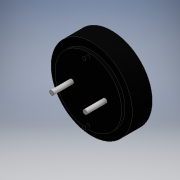
# Autodesk Inventor part: BUZZER_TDK_PS12
Saved by Autodesk Inventor 2016 (Build 200138000, 138)
## iProperties
Created: 2018-08-01
Part Number: BUZZER_TDK_PS12
Material: Generic
Document SubType Name: Modeling
Designer: Luke
Density: 1 g/cm^3
Appearance: Default
Author: Luke
Autodesk Inventor part; units mm, degrees
ref_plane "YZ Plane" through (0, 0, 0) normal (1, 0, 0) x (0, 1, 0)
ref_plane "XZ Plane" through (0, 0, 0) normal (0, 1, 0) x (-1, 0, 0)
ref_plane "XY Plane" through (0, 0, 0) normal (0, 0, 1) x (1, 0, 0)
sketch "Sketch1" plane through (0, 0, 0) normal (0, 1, 0) x (-1, 0, 0)
  circle A0 centre (0, 0) radius 6.1
  dimension "d0" = 12.2
  constraints: 1 centre point, 1 coincident
  measures "d0" diameter of A0
extrude "Extrusion1" add sketch "Sketch1" along normal blind 3.5
sketch "Sketch2" plane through (0, 3.5, 0) normal (0, 1, 0) x (1, 0, 0)
  circle A0 centre (0, 0) radius 1.5
  dimension "d3" = 3
  constraints: 1 centre point, 1 coincident
  measures "d3" diameter of A0
extrude "Extrusion2" cut sketch "Sketch2" against normal blind 1
sketch "Sketch3" plane through (0, 0, 0) normal (0, -1, 0) x (1, 0, 0)
  circle A0 centre (0, 0) radius 5
  circle A1 centre (0, 0) radius 6.1 projected
  dimension "d6" = 10
  constraints: 1 centre point, 1 coincident
  measures "d6" diameter of A0
extrude "Extrusion3" cut sketch "Sketch3" against normal blind 0.5
sketch "Sketch4" plane through (0, 0, 0) normal (0, 1, 0) x (-1, 0, 0)
  line L0 (-8.54, 0) -> (8.54, 0) construction
  circle A0 centre (-2.5, 0) radius 0.325
  circle A1 centre (2.5, 0) radius 0.325
  line L1 (0, -8.54) -> (0, 8.54) construction
  point P0 (0, 0)
  dimension "d9" = 0.65
  dimension "d10" = 0.65
  dimension "d11" = 5
  constraints: 2 centre point, 2 point on line, 1 symmetric about line
  measures "d9" diameter of A0
  measures "d10" diameter of A1
  measures "d11" distance of A1.centre A0.centre
extrude "Extrusion4" add sketch "Sketch4" against normal blind 3
sketch "Sketch5" plane through (0, 0, 0) normal (0, -1, 0) x (1, 0, 0)
  line L0 (0, 8.54) -> (0, -8.54) construction
  line L1 (-8.54, 0) -> (8.54, 0) construction
  circle A0 centre (0, -4.5) radius 0.25
  circle A1 centre (0, 4.5) radius 0.25
  point P0 (0, 0)
  dimension "d14" = 0.5
  dimension "d15" = 0.5
  dimension "d16" = 9
  constraints: 2 centre point, 2 point on line, 1 symmetric about line
  measures "d14" diameter of A0
  measures "d15" diameter of A1
  measures "d16" distance of A1.centre A0.centre
extrude "Extrusion5" add sketch "Sketch5" along normal blind 0.6
body "Solid1"
